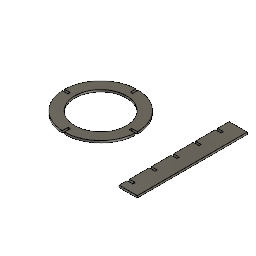
Pressfit Construction (Autodesk Fusion 360 design; units mm, degrees)
Autodesk Fusion 360 part; units mm, degrees
sketch "Sketch1" plane through (0, 0, 0) normal (0, 0, 1) x (1, 0, 0)
  line L0 (1.4478, 49.979) -> (1.4478, 41.979)
  line L1 (1.4478, 41.979) -> (-1.4522, 41.979)
  line L2 (-1.4522, 41.979) -> (-1.4522, 49.9789)
  line L3 (-49.9982, 0.4218) -> (-41.9982, 0.4353)
  line L4 (-41.9933, -2.4646) -> (-49.9393, -2.462)
  line L5 (-41.9982, 0.4353) -> (-41.9933, -2.4646)
  line L6 (-2.494, -49.9378) -> (-2.3689, -41.9972)
  line L7 (0.5311, -41.9972) -> (0.5311, -49.9972)
  line L8 (-2.3689, -41.9972) -> (0.5311, -41.9972)
  line L9 (49.9262, -2.7151) -> (41.9262, -2.7471)
  line L10 (41.9997, 0.1519) -> (49.9997, 0.184)
  line L11 (41.9262, -2.7471) -> (41.9997, 0.1519)
  circle A0 centre (0, 0) radius 35
  line L12 (100.1319, 74.6129) -> (125.1319, 74.6129)
  line L13 (125.1319, 74.6129) -> (125.1319, -75.3871)
  line L14 (125.1319, -75.3871) -> (100.1319, -75.3871)
  line L15 (100.1319, -61.4369) -> (108.1319, -61.4369)
  line L16 (108.1319, -61.4369) -> (108.1319, -64.4369)
  line L17 (108.1319, -64.4369) -> (100.1319, -64.4369)
  line L18 (100.1319, -31.4369) -> (108.1319, -31.4369)
  line L19 (108.1319, -34.3369) -> (100.1319, -34.3369)
  line L20 (108.1319, -31.4369) -> (108.1319, -34.3369)
  line L21 (100.1319, -1.4369) -> (108.1319, -1.4369)
  line L22 (108.1319, -4.3369) -> (100.1319, -4.3369)
  line L23 (108.1319, -1.4369) -> (108.1319, -4.3369)
  line L24 (100.1319, 28.5631) -> (108.1319, 28.5631)
  line L25 (108.1319, 25.6631) -> (100.1319, 25.6631)
  line L26 (108.1319, 28.5631) -> (108.1319, 25.6631)
  line L27 (100.1319, 58.5631) -> (108.1319, 58.5631)
  line L28 (108.1319, 55.6631) -> (100.1319, 55.6631)
  line L29 (108.1319, 58.5631) -> (108.1319, 55.6631)
  arc A1 (49.9997, 0.184) -> (1.4478, 49.979) centre (0, 0) ccw
  arc A2 (-1.4522, 49.9789) -> (-49.9982, 0.4218) centre (0, 0) ccw
  arc A3 (-49.9393, -2.462) -> (-2.494, -49.9378) centre (0, 0) ccw
  arc A4 (0.5311, -49.9972) -> (49.9262, -2.7151) centre (0, 0) ccw
  line L30 (100.1319, 58.5631) -> (100.1319, 74.6129)
  line L31 (100.1319, 28.5631) -> (100.1319, 55.6631)
  line L32 (100.1319, -1.4369) -> (100.1319, 25.6631)
  line L33 (100.1319, -31.4369) -> (100.1319, -4.3369)
  line L34 (100.1319, -75.3871) -> (100.1319, -64.4369)
  line L35 (100.1319, -61.4369) -> (100.1319, -34.3369)
  dimension "d6" = 70
  dimension "d7" = 25
  dimension "d8" = 150
  dimension "d9" = 8
  dimension "d10" = 3
  dimension "d15" = 100
  dimension "d23" = 2.9
  dimension "d24" = 8
  dimension "d25" = 2.9
  dimension "d26" = 8
  dimension "d27" = 8
  dimension "d28" = 2.9
  dimension "d29" = 8
  dimension "d30" = 2.9
  dimension "d31" = 8
  dimension "d32" = 2.9
  dimension "d33" = 8
  dimension "d34" = 2.9
  dimension "d35" = 8
  dimension "d36" = 2.9
  dimension "d37" = 8
  dimension "d38" = 2.9
  dimension "d39" = 8
  dimension "d42" = 15
  constraint vertical L0
  constraint horizontal L1
  constraint vertical L2
  constraint coincident A0.centre A1.centre
  constraint horizontal L12
  constraint vertical L13
  constraint horizontal L14
  constraint vertical L34
  constraint horizontal L15
  constraint vertical L16
  constraint horizontal L17
  constraint coincident L15.start L34
  constraint coincident L10.end A2
  constraint concentric A1 A2
  constraint equal L9 L10
  constraint parallel L9 L10
  constraint concentric A2 A3
  constraint coincident L7.end A3
  constraint concentric A3 A4
  constraint collinear L30 L34
  constraint collinear L31 L34
  constraint collinear L32 L34
  constraint collinear L33 L34
  constraint collinear L34 L35
  constraint equal L18 L19
  constraint equal L21 L22
  constraint equal L24 L25
  constraint equal L27 L28
  constraint concentric A0 A1
  measures "d6" diameter of A0
  measures "d7" distance of L12.start L12.end
  measures "d8" distance of L12.start L14.end
  measures "d9" distance of L15.start L15.end
  measures "d10" distance of L15.start L17.end
  measures "d15" diameter of A2
  measures "d23" distance of L0.end L1.end
  measures "d24" distance of L0.end L0.start
  measures "d25" distance of L9.end L10.start
  measures "d26" horizontal distance of L10.start L10.end
  measures "d27" distance of L3.end L3.start
  measures "d28" distance of L3.end L4.start
  measures "d29" distance of L7.start L7.end
  measures "d30" distance of L6.end L7.start
  measures "d31" distance of L27.start L27.end
  measures "d32" distance of L27.end L28.start
  measures "d33" distance of L24.start L24.end
  measures "d34" distance of L24.end L25.start
  measures "d35" distance of L21.start L21.end
  measures "d36" distance of L21.end L22.start
  measures "d37" distance of L18.start L18.end
  measures "d38" distance of L18.end L19.start
  measures "d39" distance of L16.end L17.end
  measures "d42" distance of A0 A4
extrude "Extrude1" add sketch "Sketch1" along normal blind 3 makes body 1 at (-41.4923, -7.5131, 0) makes body 2 at (119.4652, -0.7371, 0)
equation "d6 = small_circle"
equation "d7 = rec_width"
equation "d8 = rec_height"
equation "d15 = big_circle"
equation "kerf = 0.1 mm"
equation "big_circle = 100 mm"
equation "small_circle = 70 mm"
equation "slot_height = 8 mm"
equation "material_thickness = 3 mm"
equation "slot_width = material_thickness - kerf"
equation "d23 = slot_width"
equation "d24 = slot_height"
equation "d25 = slot_width"
equation "d26 = slot_height"
equation "d27 = slot_height"
equation "d28 = slot_width"
equation "d29 = slot_height"
equation "d30 = slot_width"
equation "d31 = slot_height"
equation "d32 = slot_width"
equation "d33 = slot_height"
equation "d34 = slot_width"
equation "d35 = slot_height"
equation "d36 = slot_width"
equation "d37 = slot_height"
equation "d38 = slot_width"
equation "rec_height = 150 mm"
equation "rec_width = 25 mm"
